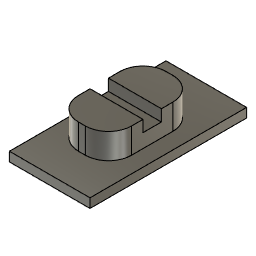
switch (Autodesk Fusion 360 design; units mm, degrees)
Autodesk Fusion 360 part; units mm, degrees
sketch "草图1" plane through (0, 0, 0) normal (0, 0, 1) x (1, 0, 0)
  line L0 (0.5, 0.5, 1.2) -> (7.5, 0.5, 1.2)
  line L1 (7.5, 0.5, 1.2) -> (7.5, 14.1, 1.2)
  line L2 (7.5, 14.1, 1.2) -> (0.5, 14.1, 1.2)
  line L3 (0.5, 14.1, 1.2) -> (0.5, 0.5, 1.2)
  line L4 (1.5, 3.5, 2) -> (6.1, 3.5, 2)
  line L5 (6.1, 3.5, 2) -> (6.1, 11.1, 2)
  line L6 (6.1, 11.1, 2) -> (1.5, 11.1, 2)
  line L7 (1.5, 11.1, 2) -> (1.5, 3.5, 2)
  line L8 (4.1, 3.5) -> (6.1, 3.5)
  line L9 (6.1, 3.5) -> (6.1, 6.5)
  line L10 (6.1, 6.5) -> (4.1, 6.5)
  line L11 (4.1, 6.5) -> (4.1, 3.5)
  line L12 (6.1, 8.1) -> (4.1, 8.1)
  line L13 (4.1, 8.1) -> (4.1, 11.1)
  line L14 (4.1, 11.1) -> (6.1, 11.1)
  line L15 (6.1, 11.1) -> (6.1, 8.1)
  point P0 (1.5, 3.5)
  dimension "d1" = 13.6
  dimension "d2" = 4.6
  dimension "d3" = 7.6
  constraint horizontal L8
  constraint vertical L9
  constraint horizontal L10
  constraint vertical L11
  constraint horizontal L12
  constraint vertical L13
  constraint horizontal L14
  constraint vertical L15
  measures "d2" distance of P0 L8.end
extrude "拉伸4" add sketch "草图1" along normal blind 1.2 makes body 1 at (4.7667, 5.5, 0) makes body 2 at (5.4333, 9.1, 0)
extrude "拉伸5" add sketch "草图1" along normal blind 0.8 contours L0 L1 L2 L3 in plane through (0, 0, 1.2) normal (0, 0, 1) bodies 1 2
extrude "拉伸6" add sketch "草图1" along normal blind 2.2 contours L4 L5 L6 L7 in plane through (0, 0, 2) normal (0, 0, 1) bodies 1
box "长方体基本要素2" cut length 1.6 width 9 height -1 placed x (0, 1, 0) y (-1, 0, 0) z (0, 0, 1) at (9, 6.5, 4.2) bodies 1
fillet "圆角1" radius 2 4 edges at (1.5, 3.5, 3.1) (6.1, 3.5, 3.1) (6.1, 11.1, 3.1) (1.5, 11.1, 3.1) on bodies 1
